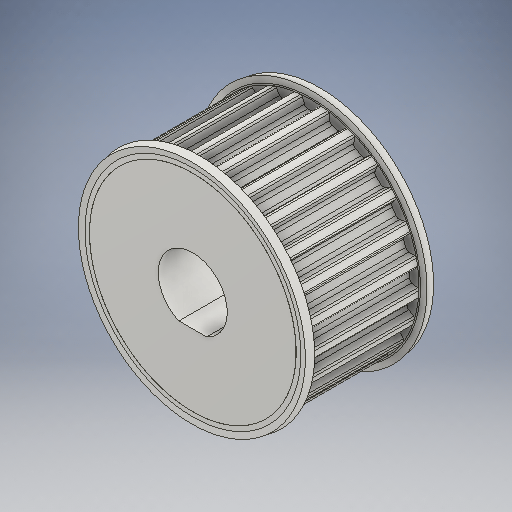
# Autodesk Inventor part: Nem_pulley
Saved by Autodesk Inventor 2025.2 (Build 292293000, 293)
## iProperties
Created: 2025-04-07
Part Number: Nem_pulley
Material: Steel
Document SubType Name: Modeling
Designer: Tiago
Density: 1 g/cm^3
Appearance: Steel
Author: Tiago
Autodesk Inventor part; units mm, degrees
ref_plane "YZ Plane" through (0, 0, 0) normal (1, 0, 0) x (0, 1, 0)
ref_plane "XZ Plane" through (0, 0, 0) normal (0, 1, 0) x (-1, 0, 0)
ref_plane "XY Plane" through (0, 0, 0) normal (0, 0, 1) x (1, 0, 0)
sketch "Pulley Sketch" plane through (0, 0, 0) normal (0, 0, 1) x (1, 0, 0)
  circle A0 centre (0, 0) radius 8.0851 construction
  circle A1 centre (0, 0) radius 7.8311
  circle A2 centre (0, 0) radius 7.1453
  line L0 (-0.6586, 7.8033) -> (-0.4191, 7.1453)
  line L1 (-0.4191, 7.1453) -> (0.4191, 7.1453)
  line L2 (0.4191, 7.1453) -> (0.6586, 7.8033)
  line L3 (0, 0) -> (0, 7.8311) construction
  point P0 (0, 7.1453)
  dimension "d0" = 16.1701
  dimension "d1" = 0.254
  dimension "d2" = 0.6858
  dimension "d3" = 40
  dimension "d4" = 0.8382
  constraints: 8 end point, 3 coincident, 3 point on circle, 2 centre point, 1 horizontal, 1 midpoint, 1 point on line, 1 vertical, 1 vertical alignment, 3 other
  measures "d0" diameter of A0
  measures "d1" radial gap between concentric circles of A0 A1
  measures "d3" angle of L2 L0
  measures "d4" distance of L0.end L1.end
extrude "Base Body" add sketch "Pulley Sketch" along normal mid plane 8 contours A2 | A1 L0 L1 L2 | L2 L1 L0 A1
extrude "Tooth" cut sketch "Pulley Sketch" along normal through all both and the other way through all contours L2 L1 L0 A1 picked at (0, 7.6004)
fillet "Tooth Fillet" radius 0.254 2 edges at (0.4191, 7.1453, 0) (-0.4191, 7.1453, 0)
fillet "Tooth Fillet" radius 0.127 4 edges at (-0.6586, 7.8033, 2) (-0.6586, 7.8033, -2) (0.6586, 7.8033, 2) (0.6586, 7.8033, -2)
pattern_circular "Teeth" count 25 over 360 about axis through (0, 0, -10) along (0, 0, 1) of "Tooth", "Tooth Fillet"
pulley flange "Left flange" diameter 15.6621 height 0.508 thickness 0.5842 bend angle 10 centre (0, 0, -4) toward (0, 0, -1)
pulley flange "Right flange" diameter 15.6621 height 0.508 thickness 0.5842 bend angle 10 centre (0, 0, 4) toward (0, 0, 1)
sketch "Sketch2" plane through (0, 0, 4.5842) normal (0, 0, 1) x (1, 0, 0)
  circle A0 centre (0, 0) radius 2.5
  circle A1 centre (0.0459, -0.0398) radius 2.5
  line L0 (0.0459, -0.0398) -> (0.0459, -2.2898)
  line L1 (0.0459, -2.2898) -> (1.1356, -2.2898)
  line L2 (1.1356, -2.2898) -> (1.1356, -2.5398)
  line L3 (0.0459, -2.2898) -> (-1.0439, -2.2898)
  line L4 (-1.0439, -2.2898) -> (-1.0439, -2.5398)
  line L5 (-1.0439, -2.5398) -> (1.1356, -2.5398)
  point P0 (-1.0034, -2.2898)
  point P1 (1.0034, -2.2898)
  dimension "d17" = 5
  dimension "d20" = 2.25
  constraints: 12 end point, 3 vertical, 2 centre point, 2 coincident, 2 horizontal, 2 point on circle, 1 perpendicular
  measures "d17" diameter of A0
  measures "d20" distance of L0.start L0.end
extrude "Extrusion3" cut sketch "Sketch2" against normal up to surface (9.1684 mm away) contours A0 L1 L3 A1 | A1 A0 picked at (1.0741, 0.4624)
sketch "Sketch3" plane through (0, 0, 4.5842) normal (0, 0, 1) x (1, 0, 0)
  circle A0 centre (0, 0) radius 8.3391
  circle A1 centre (0, 0) radius 2.5
  line L0 (1.0034, -2.2898) -> (-1.0034, -2.2898) projected
  line L1 (0, -2.2898) -> (-1.0034, -2.2898)
  line L2 (-1.0034, -2.2898) -> (1.0034, -2.2898)
  circle A2 centre (0, 0) radius 7.5
  dimension "d23" = 15
  constraints: 4 end point, 3 centre point, 3 coincident, 1 collinear, 1 horizontal, 1 midpoint
  measures "d23" diameter of A2
extrude "Extrusion4" add sketch "Sketch3" along normal blind 0.01 contours L0 A1 | A2 picked at (0.5053, -2.3422)
sketch "Sketch4" plane through (-1.0034, -2.2898, -4.5842) normal (0, 1, 0) x (1, 0, 0)
  line L0 (-6.4854, 0) -> (0, 0) projected
  line L1 (0, -9.1784) -> (0, 0) projected
  line L2 (0, -9.1784) -> (-6.1385, -9.1784) projected
  line L3 (-6.1385, -9.1784) -> (-6.1385, -9.1684) projected
  line L4 (-6.1385, -9.1684) -> (-6.4854, -9.1684) projected
  line L5 (-6.4854, -8.5842) -> (-6.4854, -0.5842) projected
  line L6 (0, 0) -> (2.0068, 0) projected
  line L7 (2.0068, 0) -> (2.0068, -9.1784) projected
  line L8 (2.0068, -9.1784) -> (0, -9.1784) projected
  line L9 (2.0068, 0) -> (8.4922, 0) projected
  line L10 (8.4922, -0.5842) -> (8.4922, -8.5842) projected
  line L11 (8.4922, -9.1684) -> (8.1453, -9.1684) projected
  line L12 (8.1453, -9.1684) -> (8.1453, -9.1784) projected
  line L13 (8.1453, -9.1784) -> (2.0068, -9.1784) projected
  line L14 (0, -9.1784) -> (0, 0)
  line L15 (0, 0) -> (2.0068, 0)
  line L16 (2.0068, -9.1784) -> (2.0068, 0)
  line L17 (0, -9.1784) -> (2.0068, -9.1784)
  point P0 (1.0034, -4.5842)
  constraints: 8 end point, 2 collinear, 2 perpendicular, 16 other
extrude "Extrusion5" cut sketch "Sketch4" against normal blind 0.0001
equation "\"d1\" = da_a"
equation "\"d2\" = da_hg"
equation "\"d3\" = 2 * da_fi"
equation "\"d4\" = da_bw"
equation "\"d5\" = da_bf"
equation "\"d7\" = da_bf"
equation "\"d9\" = da_rb"
equation "\"d10\" = da_rt"
equation "\"da_pb\" = 2.032"
equation "\"da_fi\" = 20deg"
equation "\"da_hg\" = 0.6858"
equation "\"da_bw\" = 0.8382"
equation "\"da_rb\" = 0.254"
equation "\"da_rt\" = 0.127"
equation "\"da_a\" = 0.254"
equation "\"da_bf\" = 8"
equation "\"da_wf\" = 0.5842"
equation "\"da_hf\" = 0.508"
body "Solid1"
